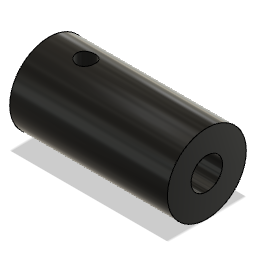
motor connector v2 v3 (Autodesk Fusion 360 design; units mm, degrees)
Autodesk Fusion 360 part; units mm, degrees
sketch "Sketch1" plane through (0, 0, 0) normal (1, 0, 0) x (0, 0, -1)
  circle A0 centre (0, 0) radius 3
  circle A1 centre (0, 0) radius 7.5
  dimension "d1" = 6
  dimension "d2" = 15
  constraint coincident A0.centre A1.centre
  measures "d1" diameter of A0
  measures "d2" diameter of A1
extrude "Extrude1" add sketch "Sketch1" against normal blind 15
sketch "Sketch2" plane through (-15, 0, 0) normal (-1, 0, 0) x (0, 0, 1)
  circle A0 centre (0, 0) radius 7.5
  circle A1 centre (0, 0) radius 3.25
  circle A2 centre (0, 0) radius 7.5
  dimension "d5" = 6.5
  constraint concentric A1 A2
  measures "d5" diameter of A1
extrude "Extrude2" add sketch "Sketch2" along normal blind 15
sketch "Sketch3" plane through (0, 0, 0) normal (0, 1, 0) x (1, 0, 0)
  line L0 (-30, 7.5) -> (-30, -7.5)
  line L1 (0, -7.5) -> (0, 7.5)
  circle A0 centre (-23, 0) radius 1.75
  point P0 (-23, 0)
  dimension "d8" = 30
  constraint coincident P0 A0.centre
  measures "d8" distance of L0 L1
extrude "Extrude3" cut sketch "Sketch3" along normal mid plane 38
